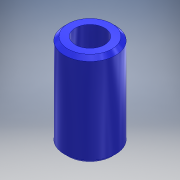
# Autodesk Inventor part: acople
Saved by Autodesk Inventor 2018 (Build 220112000, 112)
## iProperties
Created: 2019-05-16
Part Number: acople
Material: Generic
Document SubType Name: Modeling
Designer: JLVega003
Density: 1 g/cm^3
Appearance: Blue - Wall Paint - Glossy
Author: JLVega003
Autodesk Inventor part; units mm, degrees
ref_plane "YZ Plane" through (0, 0, 0) normal (1, 0, 0) x (0, 1, 0)
ref_plane "XZ Plane" through (0, 0, 0) normal (0, 1, 0) x (-1, 0, 0)
ref_plane "XY Plane" through (0, 0, 0) normal (0, 0, 1) x (1, 0, 0)
sketch "Sketch1" plane through (0, 0, 0) normal (0, 1, 0) x (-1, 0, 0)
  line L0 (-4, -12.7) -> (-7, -12.7)
  line L1 (-7, -12.7) -> (-7, 12.7)
  line L2 (-7, 12.7) -> (-4, 12.7)
  line L3 (-4, 12.7) -> (-4, -12.7)
  line L4 (0, -17.78) -> (0, 17.78) construction
  line L5 (1.4, 0) -> (-8.4, 0) construction
  point P0 (0, 0)
  point P1 (-4, 0)
  dimension "d0" = 8
  dimension "d1" = 14
  dimension "d2" = 25.4
  constraints: 8 end point, 2 parallel, 1 horizontal, 1 midpoint, 1 perpendicular, 1 point on line
  measures "d0" diameter of L3 L4
  measures "d1" diameter of L1 L4
  measures "d2" distance between parallel lines of L2 L0
revolve "Revolution1" add sketch "Sketch1" angle 360 about axis through (0, 0, -10) along (0, 0, 1)
chamfer "Chamfer1" distance 1 angle 45 2 edges at (-7, 0, 12.7) (-7, 0, -12.7)
body "Solid1"
